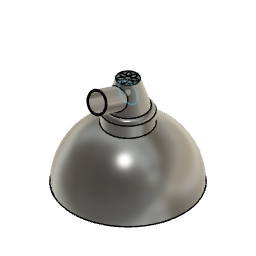
lamp v4 (Autodesk Fusion 360 archive; units mm, degrees)
design "BULB HOLDER"
Autodesk Fusion 360 part; units mm, degrees
note: some values were not read from the file. Chosen so that the rebuilt part matches the saved one: where a step ends; which pieces of a blend or face edit are solid.
sketch "Sketch1" plane through (0, 0, 0) normal (0, 1, 0) x (1, 0, 0)
  line L0 (-100, 0) -> (0, 0)
  line L1 (0, 0) -> (0, -100)
  arc A0 (-100, 0) -> (0, -100) centre (0, 0) ccw
  dimension "d1" = 200
  constraint coincident L0.end L1.start
  constraint horizontal L0
  constraint perpendicular L0 L1
  measures "d1" diameter of A0
revolve "Revolve1" add sketch "Sketch1" angle 360 about axis through (0, 0, 0) along (0, 0, 1)
shell "Shell1" thickness 2 removed faces 1 at (27.1036, 4.9681, 0)
sketch "Sketch2" plane through (0, 0, 0) normal (0, 0, 1) x (1, 0, 0)
ref_plane "WorkPlane1" through (0, 0, 100) normal (0, 0, 1) x (1, 0, 0)
sketch "Sketch3" plane through (0, 0, 100) normal (0, 0, 1) x (1, 0, 0)
  circle A0 centre (0, 0) radius 36.0555
  constraint coincident A0.centre origin
extrude "Extrude1" add sketch "Sketch3" along normal up to surface end surface at (-49.5722, 85.8616, 13.0526)
extrude "Extrude2" add 1 faces at (-5.9453, 7.96, 100) along direction (0, 0, 1) blind 20
fillet "Fillet1" radius 7.5 1 edges at (-33.6155, -13.0382, 120)
sketch "Sketch4" plane through (0, 0, 0) normal (0, 1, 0) x (1, 0, 0)
  line L0 (-30, -120) -> (-15.9595, -162.1214)
  line L1 (-15.9595, -162.1214) -> (0, -162.1214)
  line L2 (0, -162.1214) -> (0, -120)
  line L3 (0, -120) -> (-30, -120)
  line L4 (0, -167.5879) -> (0, -107.2604) construction
  constraint horizontal L1
  constraint perpendicular L1 L2
  constraint perpendicular L2 L3
  constraint perpendicular L3 L4
revolve "Revolve2" add sketch "Sketch4" angle 360 about axis through (0, 0, 167.5879) along (0, 0, -1)
sketch "Sketch5" plane through (0, 0, 0) normal (0, 1, 0) x (1, 0, 0)
  circle A0 centre (0, -140) radius 17
  dimension "d12" = 34
  measures "d12" diameter of A0
ref_plane "WorkPlane2" through (0, -22.9798, 141.0607) normal (0, -0.948683, 0.316228) x (1, 0, 0)
sketch "Sketch6" plane through (0, -22.9798, 141.0607) normal (0, -0.948683, 0.316228) x (1, 0, 0)
  circle A0 centre (0.1328, 0.289) radius 17
  dimension "d14" = 34
  measures "d14" diameter of A0
extrude "Extrude3" add sketch "Sketch6" along normal up to near side of body 1
extrude "Extrude4" add 1 faces at (-3.0649, -23.2323, 140.3032) along direction (0, -0.948683, 0.316228) blind 30
sketch "Sketch7" plane through (0, 0, 0) normal (0, 1, 0) x (-1, 0, 0)
sketch "Sketch8" plane through (0, 0, 162.1214) normal (0, 0, 1) x (-1, 0, 0)
  circle A0 centre (0, 0) radius 15.9595
ref_plane "WorkPlane3" through (0, 0, 162.1214) normal (0, 0, 1) x (-1, 0, 0)
sketch "Sketch9" plane through (0, 0, 162.1214) normal (0, 0, 1) x (-1, 0, 0)
  ellipse E0 centre (5.6177, -7.0427) end of major axis (2.5253, -3.1137) minor radius 3.2533
  line L0 (8.7101, -10.9717) -> (2.5253, -3.1137)
  line L1 (8.1742, -5.0306) -> (3.0612, -9.0548)
  ellipse E1 centre (9.0088, 0.0011) end of major axis (4.0089, 0.033) minor radius 3.2533
  ellipse E2 centre (5.616, 7.044) end of major axis (2.4737, 3.1549) minor radius 3.2533
  ellipse E3 centre (-2.0057, 8.7827) end of major axis (-0.9243, 3.901) minor radius 3.2533
  ellipse E4 centre (-8.1171, 3.9078) end of major axis (-3.6262, 1.7096) minor radius 3.2533
  ellipse E5 centre (-8.1162, -3.9097) end of major axis (-3.5975, -1.7691) minor radius 3.2533
  ellipse E6 centre (-2.0036, -8.7831) end of major axis (-0.8598, -3.9157) minor radius 3.2533
  dimension "d21" = 360
  constraint coincident E0 L0.start
  constraint coincident E0 L0.end
  constraint coincident E0 L1.start
  constraint coincident E0 L1.end
extrude "Extrude5" cut sketch "Sketch9" against normal blind 5
delete_face "DeleteFace1" 1 faces at (17.1326, -39.6265, 147.0076)
ref_plane "WorkPlane4" through (0, -22.9798, 141.0607) normal (0, -0.948683, 0.316228) x (1, 0, 0)
sketch "Sketch10" plane through (0, -22.9798, 141.0607) normal (0, -0.948683, 0.316228) x (1, 0, 0)
  circle A0 centre (0, 0) radius 17
  circle A1 centre (0, 0) radius 15
  dimension "d25" = 34
  dimension "d26" = 30
  constraint coincident A0.centre A1.centre
  measures "d25" diameter of A0
  measures "d26" diameter of A1
extrude "Extrude6" add sketch "Sketch10" against normal blind 5.101
extrude "Extrude7" add 1 faces at (-1.5898, -28.1071, 125.6786) along direction (0, -0.948683, 0.316228) blind 35
